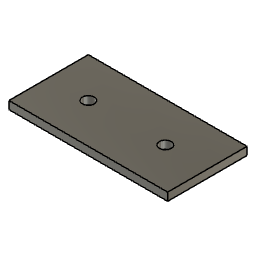
VL53LXX-V2_Holder v1 (Autodesk Fusion 360 design; units mm, degrees)
Autodesk Fusion 360 part; units mm, degrees
sketch "Esquisse1" plane through (0, 0, 0) normal (0, 0, 1) x (1, 0, 0)
  line L0 (0, 0) -> (40, 0)
  line L1 (40, 0) -> (40, 20)
  line L2 (40, 20) -> (0, 20)
  line L3 (0, 20) -> (0, 0)
  circle A0 centre (10.0023, 10.0061) radius 1.5
  circle A1 centre (29.4023, 10.0056) radius 1.5
  dimension "d1" = 3
  dimension "d2" = 3
  dimension "d3" = 19.4
  constraint horizontal L0
  constraint vertical L1
  constraint horizontal L2
  constraint vertical L3
  constraint coincident L0.start L3.end
  measures "d1" diameter of A0
  measures "d2" diameter of A1
  measures "d3" distance of A0.centre A1.centre
extrude "Extrusion1" add sketch "Esquisse1" along normal blind 2
equation "d3 = 16.4 mm + 3 mm"
